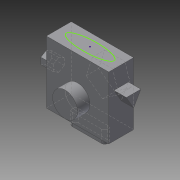
# Autodesk Inventor part: Demo-Status-0.3
Saved by Autodesk Inventor 2015 (Build 190159000, 159)
## iProperties
Created: 2017-05-12
Part Number: Demo-Status-0.3
Material: Generisch
Document SubType Name: Modeling
Designer: jensp
Density: 1 g/cm^3
Appearance: Vorgabe
Author: jensp
Autodesk Inventor part; units mm, degrees
ref_plane "YZ Plane" through (0, 0, 0) normal (1, 0, 0) x (0, 1, 0)
ref_plane "XZ Plane" through (0, 0, 0) normal (0, 1, 0) x (-1, 0, 0)
ref_plane "XY Plane" through (0, 0, 0) normal (0, 0, 1) x (1, 0, 0)
sketch "Rechteck" plane through (0, 0, 0) normal (0, 0, 1) x (1, 0, 0)
  line L0 (-5, 2) -> (5, 2)
  line L1 (5, 2) -> (5, -2)
  line L2 (5, -2) -> (-5, -2)
  line L3 (-5, -2) -> (-5, 2)
  point P0 (0, 0)
  dimension "d0" = 5
  dimension "d1" = 10
  dimension "d2" = 4
  dimension "d3" = 2
  constraints: 8 end point, 2 parallel, 1 horizontal, 1 perpendicular
  measures "d0" distance from line of point (0, 0) L3
  measures "d1" distance of L1.end L2.end
  measures "d2" distance of L0.end L1.end
  measures "d3" distance from line of point (0, 0) L2
extrude "Extrusion1" add sketch "Rechteck" along normal blind 10
sketch "Kreis" plane through (-5, -2, 0) normal (0, -1, 0) x (1, 0, 0)
  circle A0 centre (5, 4) radius 2
  point P0 (5, 0)
  dimension "d6" = 4
  constraints: 1 centre point
  measures "d6" diameter of A0
extrude "Extrusion2" add sketch "Kreis" along normal blind 2
sketch "Dreieck" plane through (5, -2, 0) normal (1, 0, 0) x (0, 0, -1)
  line L0 (-5.0135, 2) -> (-7.0323, 0.8344)
  line L1 (-7.0323, 0.8344) -> (-7.0323, 3.1656)
  line L2 (-7.0323, 3.1656) -> (-5.0135, 2)
  point P0 (0, 2)
  point P1 (-6.3594, 2)
  constraints: 6 end point, 7 other
extrude "Extrusion3" add sketch "Dreieck" along normal blind 2
sketch "Pentagon" plane through (-5, 2, 0) normal (0, 1, 0) x (1, 0, 0)
  line L0 (5, -1.7907) -> (7.6131, -3.6893)
  line L1 (7.6131, -3.6893) -> (6.615, -6.7612)
  line L2 (6.615, -6.7612) -> (3.385, -6.7612)
  line L3 (3.385, -6.7612) -> (2.3869, -3.6893)
  line L4 (2.3869, -3.6893) -> (5, -1.7907)
  point P0 (5, 0)
  point P1 (5, -4.5383)
  constraints: 10 end point, 11 other
extrude "Extrusion4" add sketch "Pentagon" along normal blind 2
sketch "Hexagon" plane through (-5, -2, 0) normal (-1, 0, 0) x (0, 0, 1)
  line L0 (6.0229, 2) -> (5.5093, 1.1104)
  line L1 (5.5093, 1.1104) -> (4.4821, 1.1104)
  line L2 (4.4821, 1.1104) -> (3.9685, 2)
  line L3 (3.9685, 2) -> (4.4821, 2.8896)
  line L4 (4.4821, 2.8896) -> (5.5093, 2.8896)
  line L5 (5.5093, 2.8896) -> (6.0229, 2)
  point P0 (0, 2)
  point P1 (4.9957, 2)
  constraints: 12 end point, 13 other
extrude "Extrusion5" add sketch "Hexagon" along normal blind 2
sketch "Ellipse" plane through (0, 0, 10) normal (0, 0, 1) x (1, 0, 0)
  ellipse E0 centre (0, 0) end of major axis (3.8358, 0) minor radius 1.1104
  constraints: 1 coincident, 2 other
sketch "Nase" plane through (0, 0, 0) normal (0, 0, -1) x (-1, 0, 0)
  line L0 (2.3535, 0) -> (-2.3535, 0) construction
  line L1 (2.3535, 0.5) -> (-2.3535, 0.5)
  line L2 (-2.3535, -0.5) -> (2.3535, -0.5)
  arc A0 (2.3535, -0.5) -> (2.3535, 0.5) centre (2.3535, 0) ccw
  arc A1 (-2.3535, 0.5) -> (-2.3535, -0.5) centre (-2.3535, 0) ccw
  point P0 (0, 0)
  dimension "d17" = 1
  constraints: 8 end point, 4 point on circle, 4 tangent, 2 centre point, 1 horizontal, 1 midpoint, 1 parallel
  measures "d17" diameter of A1
extrude "Extrusion7" add sketch "Nase" along normal blind 2
